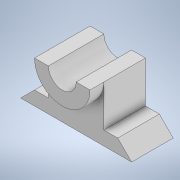
# Autodesk Inventor part: 零件1
Saved by Autodesk Inventor 2020 (Build 240168000, 168)
## iProperties
Created: 2020-09-19
Part Number: 零件1
Material: 一般
Document SubType Name: Modeling
Designer: User
Density: 1 g/cm^3
Appearance: 預設
Author: User
Autodesk Inventor part; units mm, degrees
ref_plane "YZ Plane" through (0, 0, 0) normal (1, 0, 0) x (0, 1, 0)
ref_plane "XZ Plane" through (0, 0, 0) normal (0, 1, 0) x (-1, 0, 0)
ref_plane "XY Plane" through (0, 0, 0) normal (0, 0, 1) x (1, 0, 0)
sketch "草圖1" plane through (0, 0, 0) normal (0, 0, 1) x (1, 0, 0)
  line L0 (0, 0) -> (80, 0)
  arc A0 (30, 40) -> (50, 40) centre (40, 40) ccw
  arc A1 (20, 40) -> (60, 40) centre (40, 40) ccw
  line L1 (20, 40) -> (20, 10)
  line L2 (20, 10) -> (10, 10)
  line L3 (10, 10) -> (0, 0)
  line L4 (60, 40) -> (60, 10)
  line L5 (60, 10) -> (70, 10)
  line L6 (70, 10) -> (80, 0)
  line L7 (60, 40) -> (50, 40)
  line L8 (30, 40) -> (20, 40)
  constraints: 18 end point, 4 point on circle, 3 perpendicular, 2 centre point, 2 parallel, 1 coincident, 1 horizontal, 1 tangent
extrude "擠出1" add sketch "草圖1" along normal blind 40 contours L8 A0 L7 A1
extrude "擠出2" add sketch "草圖1" along normal blind 30 contours L3 L2 L1 A1 L4 L5 L6 L0
